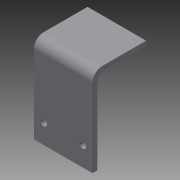
# Autodesk Inventor part: upper pulley mount
Saved by Autodesk Inventor 2013 (Build 170138000, 138)
## iProperties
Created: 2013-01-20
Part Number: upper pulley mount
Material: Generic
Document SubType Name: Sheet Metal
Designer: Arpan
Density: 1 g/cm^3
Sheet Metal Rule: Default
Author: Arpan
Autodesk Inventor part; units mm, degrees
ref_plane "YZ Plane" through (0, 0, 0) normal (1, 0, 0) x (0, 1, 0)
ref_plane "XZ Plane" through (0, 0, 0) normal (0, 1, 0) x (-1, 0, 0)
ref_plane "XY Plane" through (0, 0, 0) normal (0, 0, 1) x (1, 0, 0)
sketch "Sketch1" plane through (0, 0, 0) normal (0, 0, 1) x (1, 0, 0)
  line L0 (0, 0) -> (-38.1, 0)
  line L1 (0, 0) -> (0, 50.8)
  line L2 (0, 50.8) -> (-38.1, 50.8)
  line L3 (-38.1, 50.8) -> (-38.1, 0)
  line L4 (-38.1, 50.8) -> (-31.75, 50.8)
  line L5 (-31.75, 50.8) -> (-31.75, 12.7)
  line L6 (0, 50.8) -> (-6.35, 50.8)
  line L7 (-6.35, 50.8) -> (-6.35, 12.7)
  circle A0 centre (-31.75, 12.7) radius 2.1463
  circle A1 centre (-6.35, 12.7) radius 2.1463
  dimension "d0" = 38.1
  dimension "d1" = 50.8
  dimension "d2" = 6.35
  dimension "d3" = 38.1
  dimension "d4" = 6.35
  dimension "d5" = 4.2926
  dimension "d6" = 4.2926
  dimension "d7" = 38.1
  measures "d0" distance of L0.start L0.end
  measures "d1" distance of L0.start L1.end
  measures "d2" distance of L2.end L4.end
  measures "d3" distance of L4.end L5.end
  measures "d4" distance of L1.end L6.end
  measures "d5" diameter of A0
  measures "d6" diameter of A1
  measures "d7" distance of L6.end L7.end
extrude "Plate1" add sketch "Sketch1" along normal blind 3.175
sketch "Sketch2" plane through (0, 53.975, -3.175) normal (0, 1, 0) x (-1, 0, 0)
  line L0 (38.1, 0) -> (0, 0)
  line L1 (0, 0) -> (0, -28.575)
  line L2 (0, -28.575) -> (38.1, -28.575)
  line L3 (38.1, -28.575) -> (38.1, 0)
  constraints: 6 end point, 1 horizontal, 1 perpendicular, 1 vertical
edge flange "Flange1" height 34.925 angle 90 thickness 3.175 bend radius 3.175 thickness toward (0, 1, 0) relief straight relief width 3.175 relief depth 1.5875 corner gap 3.175 corner form 0 edges at (-34.925, 50.8, 0) (-3.175, 50.8, 0) (-19.05, 50.8, 0) wall of the first edge with corners at (-38.1, 53.975, -3.175) (0, 53.975, -3.175) (0, 53.975, -31.75) (-38.1, 53.975, -31.75)
bend "Bend1"
corner "Corner1"
equation "\"d9\" = BendReliefWidth"
equation "\"d10\" = BendReliefDepth"
equation "\"d11\" = MinimumRemnant"
equation "\"d12\" = BendRadius"
equation "\"d15\" = BendRadius"
equation "\"d16\" = CornerReliefSize"
equation "\"d17\" = GapSize"
equation "\"d18\" = JacobiRadiusSize"
equation "\"BendRadius\" = Thickness"
equation "\"BendReliefWidth\" = Thickness"
equation "\"BendReliefDepth\" = 0.5 * Thickness"
equation "\"CornerReliefSize\" = 4 * Thickness"
equation "\"MinimumRemnant\" = 2 * Thickness"
equation "\"TransitionRadius\" = BendRadius"
equation "\"JacobiRadiusSize\" = BendRadius"
equation "\"GapSize\" = Thickness"
equation "\"d8\" = BendRadius"
equation "\"Thickness\" = 3.175"
body "Solid1"
